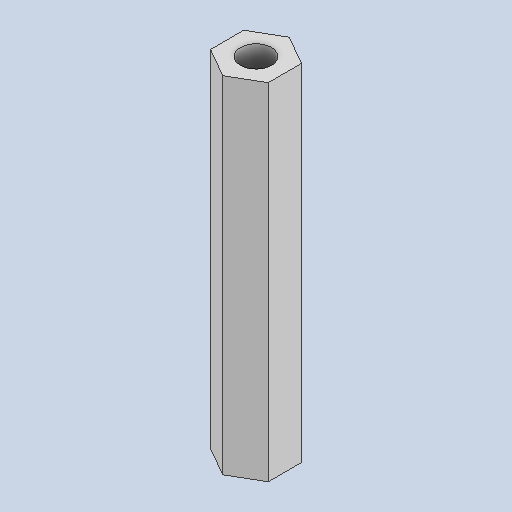
# Autodesk Inventor part: Part4
Saved by Autodesk Inventor 2024 (Build 280153000, 153)
## iProperties
Created: 2023-09-18
Part Number: Part4
Material: Generic
Document SubType Name: Modeling
Designer: Robodox
Density: 1 g/cm^3
Appearance: Default
Author: Robodox
Autodesk Inventor part; units mm, degrees
ref_plane "YZ Plane" through (0, 0, 0) normal (1, 0, 0) x (0, 1, 0)
ref_plane "XZ Plane" through (0, 0, 0) normal (0, 1, 0) x (-1, 0, 0)
ref_plane "XY Plane" through (0, 0, 0) normal (0, 0, 1) x (1, 0, 0)
sketch "Sketch1" plane through (0, 0, 0) normal (0, 1, 0) x (-1, 0, 0)
  line L0 (3.1805, -1.8236) -> (0.011, -3.6662)
  line L1 (0.011, -3.6662) -> (-3.1695, -1.8426)
  line L2 (-3.1695, -1.8426) -> (-3.1805, 1.8236)
  line L3 (-3.1805, 1.8236) -> (-0.011, 3.6662)
  line L4 (-0.011, 3.6662) -> (3.1695, 1.8426)
  line L5 (3.1695, 1.8426) -> (3.1805, -1.8236)
  circle A0 centre (0, 0) radius 1.7145
  dimension "d0" = 6.35
  dimension "d1" = 3.429
  constraints: 12 end point, 2 coincident, 1 centre point, 13 other
  measures "d0" distance between parallel lines of L2 L5
  measures "d1" diameter of A0
extrude "Extrusion1" add sketch "Sketch1" along normal blind 38.1
body "Solid1"
